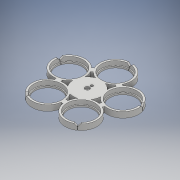
# Autodesk Inventor part: FilterWheel-2inch-5pos
Saved by Autodesk Inventor 2017 (Build 210142000, 142)
## iProperties
Created: 2022-04-07
Part Number: FilterWheel-2inch-5pos
Material: Generic
Document SubType Name: Modeling
Designer: Nikita
Density: 1 g/cm^3
Appearance: Default
Author: Nikita
Autodesk Inventor part; units mm, degrees
ref_plane "YZ Plane" through (0, 0, 0) normal (1, 0, 0) x (0, 1, 0)
ref_plane "XZ Plane" through (0, 0, 0) normal (0, 1, 0) x (-1, 0, 0)
ref_plane "XY Plane" through (0, 0, 0) normal (0, 0, 1) x (1, 0, 0)
sketch "Sketch1" plane through (0, 0, 0) normal (0, 0, 1) x (1, 0, 0)
  arc A0 (-0.4512, 77.997) -> (0.5077, 77.9956) centre (-0.0102, 50) ccw
  arc A1 (-0.4697, 74.7457) -> (0.4892, 74.745) centre (-0.0102, 50) ccw
  arc A2 (-0.4796, 72.9952) -> (0.4793, 72.9948) centre (-0.0102, 50) ccw
  line L0 (0.5077, 77.9956) -> (0.4793, 72.9948)
  line L1 (-0.4697, 74.7457) -> (-0.4512, 77.997)
  line L2 (-0.4796, 72.9952) -> (-0.4697, 74.7457)
  arc A3 (-74.3189, 23.6733) -> (-74.0214, 24.5848) centre (-47.556, 15.4411) ccw
  arc A4 (-71.2326, 22.651) -> (-70.9355, 23.5627) centre (-47.556, 15.4411) ccw
  arc A5 (-69.5708, 22.1006) -> (-69.2741, 23.0125) centre (-47.556, 15.4411) ccw
  line L3 (-74.0214, 24.5848) -> (-69.2741, 23.0125)
  line L4 (-71.2326, 22.651) -> (-74.3189, 23.6733)
  line L5 (-69.5708, 22.1006) -> (-71.2326, 22.651)
  arc A6 (-45.4804, -63.3661) -> (-46.2554, -62.8014) centre (-29.381, -40.4568) ccw
  arc A7 (-43.5545, -60.7466) -> (-44.3298, -60.1824) centre (-29.381, -40.4568) ccw
  arc A8 (-42.5175, -59.3363) -> (-43.293, -58.7723) centre (-29.381, -40.4568) ccw
  line L6 (-46.2554, -62.8014) -> (-43.293, -58.7723)
  line L7 (-43.5545, -60.7466) -> (-45.4804, -63.3661)
  line L8 (-42.5175, -59.3363) -> (-43.5545, -60.7466)
  arc A9 (46.2105, -62.8357) -> (45.434, -63.3982) centre (29.3975, -40.4449) ccw
  arc A10 (44.3144, -60.1945) -> (43.5382, -60.7575) centre (29.3975, -40.4449) ccw
  arc A11 (43.2935, -58.7725) -> (42.5175, -59.3357) centre (29.3975, -40.4449) ccw
  line L9 (45.434, -63.3982) -> (42.5175, -59.3357)
  line L10 (44.3144, -60.1945) -> (46.2105, -62.8357)
  line L11 (43.2935, -58.7725) -> (44.3144, -60.1945)
  arc A12 (74.0401, 24.5315) -> (74.3351, 23.6192) centre (47.5497, 15.4606) ccw
  arc A13 (70.9423, 23.5444) -> (71.2379, 22.6322) centre (47.5497, 15.4606) ccw
  arc A14 (69.2744, 23.0129) -> (69.5703, 22.1008) centre (47.5497, 15.4606) ccw
  line L12 (74.3351, 23.6192) -> (69.5703, 22.1008)
  line L13 (70.9423, 23.5444) -> (74.0401, 24.5315)
  line L14 (69.2744, 23.0129) -> (70.9423, 23.5444)
  circle A15 centre (0, 0) radius 24.9
  circle A16 centre (0, 0) radius 1.5
  circle A17 centre (0, 8) radius 1.25
  circle A18 centre (0, -40.4449) radius 4.5
  circle A19 centre (38.4653, -12.4981) radius 4.5
  circle A20 centre (23.7729, 32.7206) radius 4.5
  circle A21 centre (-23.7729, 32.7206) radius 4.5
  circle A22 centre (-38.4653, -12.4981) radius 4.5
  point P0 (0, 77.029)
  point P1 (-73.2589, 23.8033)
  point P2 (-45.2765, -62.3177)
  point P3 (45.2765, -62.3177)
  point P4 (73.2589, 23.8033)
  dimension "d5" = 50
  dimension "d8" = 360
  dimension "d10" = 3
  dimension "d11" = 2.5
  dimension "d14" = 24.75
  dimension "d20" = 9
  dimension "d21" = 23
  dimension "d24" = 360
  constraints: 30 end point, 30 point on circle, 23 centre point, 12 coincident, 5 point on line, 2 parallel, 92 other
  measures "d5" distance of point (0, 0) A1.centre
  measures "d10" diameter of A16
  measures "d11" diameter of A17
  measures "d14" radius of A1
  measures "d20" diameter of A18
  measures "d21" radius of A2
extrude "Extrusion1" add sketch "Sketch1" along normal blind 10 contours L1 A1 L0 A0 A20 A15 A21 | A21 A0 | A21 A3 A15 A22 L4 A4 L3 | A3 A21 | A15 A0 | A0 A15 A12 A9 A6 A3 | A3 A15 | A0 A20 | A15 A12 | A12 A20 L13 A13 L12 A19 A15 | A20 A12 | A3 A22 | A15 A6 A18 L7 A7 L6 A22 | A6 A15 | A19 A12 | A15 A9 | A9 A19 L10 A10 L9 A18 A15 | A22 A6 | A9 A19 | A6 A18 | A18 A9
sketch "Sketch2" plane through (0, 0, 10) normal (0, 0, 1) x (1, 0, 0)
  circle A0 centre (0, 0) radius 4.05
  circle A1 centre (0, 8) radius 1.25 projected
  circle A2 centre (0, 8) radius 2.25
  dimension "d15" = 8.1
  dimension "d35" = 4.5
  constraints: 2 centre point, 2 coincident
  measures "d15" diameter of A0
  measures "d35" diameter of A2
extrude "Extrusion2" cut sketch "Sketch2" against normal blind 3 contours A0
extrude "Extrusion3" add sketch "Sketch1" along normal blind 3 contours L2 A2 L0 A1 | A4 L5 A5 L3 | L14 A14 L12 A13 | A7 L8 A8 L6 | L11 A11 L9 A10
extrude "Extrusion4" add sketch "Sketch1" along normal blind 10 contours A21 A0 | A0 A21 A3 | A3 A21 | A20 A12 A0 | A0 A20 | A20 A12 | A22 A6 A3 | A3 A22 | A19 A12 | A12 A19 A9 | A22 A6 | A9 A19 | A18 A9 A6 | A6 A18 | A18 A9
sketch "Sketch3" plane through (0, 0, 0) normal (0, 0, -1) x (-1, 0, 0)
  circle A0 centre (0, 0) radius 1.5 projected
  circle A1 centre (0, 0) radius 4.05
  circle A2 centre (0, 8) radius 1.25 projected
  circle A3 centre (0, 8) radius 2.25
  dimension "d28" = 8.1
  dimension "d29" = 4.5
  constraints: 2 centre point, 2 coincident
  measures "d28" diameter of A1
  measures "d29" diameter of A3
extrude "Extrusion5" cut sketch "Sketch3" against normal blind 3
chamfer "Chamfer1" distance 4 angle 45 10 edges at (-72.4784, 24.0738, 10) (-72.7758, 23.1621, 10) (-0.4604, 76.3713, 10) (0.4984, 76.3703, 10) (72.4912, 24.0379, 10) (72.7865, 23.1257, 10) (45.2625, -61.5151, 10) (44.4861, -62.0779, 10) (-45.2926, -61.4919, 10) (-44.5175, -62.0564, 10)
extrude "Extrusion6" cut sketch "Sketch2" against normal blind 3 contours A2
body "Solid1"
